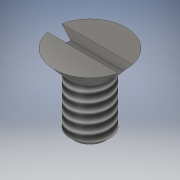
# Autodesk Inventor part: 6-32x0.25 Slotted Flathead
Saved by Autodesk Inventor 2018 (Build 220112000, 112)
## iProperties
Created: 2018-05-01
Part Number: 6-32x0.25 Slotted Flathead
Material: Stainless Steel, 440C
Document SubType Name: Modeling
Designer: Rich
Density: 7.75 g/cm^3
Appearance: Semi-Polished
Author: Rich
Autodesk Inventor part; units mm, degrees
ref_plane "YZ Plane" through (0, 0, 0) normal (1, 0, 0) x (0, 1, 0)
ref_plane "XZ Plane" through (0, 0, 0) normal (0, 1, 0) x (-1, 0, 0)
ref_plane "XY Plane" through (0, 0, 0) normal (0, 0, 1) x (1, 0, 0)
sketch "Sketch1" plane through (0, 0, 0) normal (1, 0, 0) x (0, 1, 0)
  line L0 (6.35, 0) -> (6.35, 3.175)
  line L1 (6.35, 3.175) -> (4.7137, 1.7526)
  line L2 (4.7137, 1.7526) -> (0, 1.7526)
  line L3 (0, 1.7526) -> (0, 0)
  line L4 (0, 0) -> (6.35, 0)
  line L5 (6.35, 0) -> (6.35, -3.175) construction
  line L6 (6.35, -3.175) -> (4.7137, -1.7526) construction
  line L7 (4.7137, -1.7526) -> (0, -1.7526) construction
  line L8 (0, -1.7526) -> (0, 0) construction
  dimension "d0" = 6.35
  dimension "d1" = 3.5052
  dimension "d2" = 82
  dimension "d3" = 6.35
  constraints: 18 end point, 3 perpendicular, 3 symmetric about line, 2 vertical, 1 coincident, 1 parallel
  measures "d0" distance of L5.end L0.end
  measures "d1" distance of L7.end L2.end
  measures "d2" angle of L6 L1
  measures "d3" distance of L3.end L0.start
revolve "Revolution1" add sketch "Sketch1" angle 360 about axis through (0, 0, 0) along (0, 1, 0)
sketch "Sketch2" plane through (0, 0, 0) normal (1, 0, 0) x (0, 1, 0)
  line L0 (4.7137, -1.7526) -> (4.7137, 1.7526) construction
  line L1 (6.35, -3.175) -> (6.35, 3.175) construction
  line L2 (6.35, -3.175) -> (6.35, 3.175) projected
  line L3 (6.35, 0.635) -> (5.461, 0.635)
  line L4 (5.461, 0.635) -> (5.461, -0.635)
  line L5 (5.461, -0.635) -> (6.35, -0.635)
  line L6 (6.35, -0.635) -> (6.35, 0.635)
  line L7 (6.35, 0) -> (4.7137, 0) construction
  point P0 (0, 0)
  dimension "d5" = 1.27
  dimension "d6" = 0.889
  constraints: 10 end point, 2 midpoint, 2 parallel, 1 horizontal, 1 perpendicular, 1 point on line, 1 symmetric about line
  measures "d5" distance of L5.end L3.start
  measures "d6" distance of L4.end L5.end
extrude "Extrusion1" cut sketch "Sketch2" along normal through all both and the other way through all
chamfer "Chamfer1" distance 0.381 angle 45 1 edges at (0, 0, -1.7526)
thread "Thread1" size "6-32 UNC" class "2A" standard "ANSI Unified Screw Threads" full length
body "Solid1"
